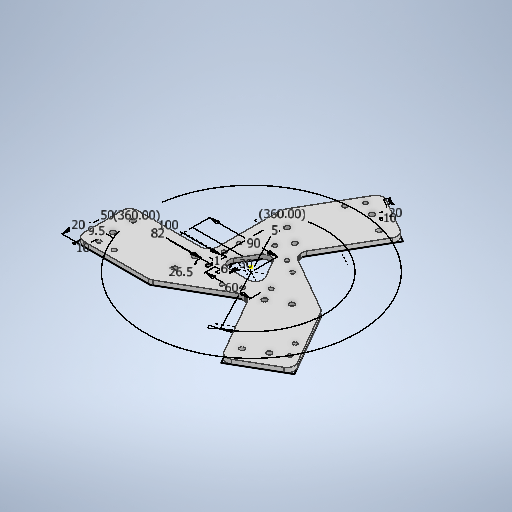
# Autodesk Inventor part: RT_FRM_MC_V3_MotorBase
Saved by Autodesk Inventor 2025.3 (Build 293356000, 356)
## iProperties
Created: 2026-09-20
Part Number: RT_FRM_MC_V3_MotorBase
Material: Generic
Document SubType Name: Modeling
Designer: louis
Density: 1 g/cm^3
Appearance: Default
Author: louis
Autodesk Inventor part; units mm, degrees
ref_plane "YZ Plane" through (0, 0, 0) normal (1, 0, 0) x (0, 1, 0)
ref_plane "XZ Plane" through (0, 0, 0) normal (0, 1, 0) x (-1, 0, 0)
ref_plane "XY Plane" through (0, 0, 0) normal (0, 0, 1) x (1, 0, 0)
sketch "Sketch1" plane through (0, 0, 0) normal (0, 0, 1) x (1, 0, 0)
  line L0 (-131, -26) -> (-49, -26) construction
  line L1 (-49, -26) -> (-49, -52.5) construction
  line L2 (-49, -52.5) -> (-131, -52.5) construction
  line L3 (-131, -52.5) -> (-131, -26) construction
  line L4 (-90, -26) -> (-90, 12) construction
  line L5 (-140, -12) -> (-40, -12) construction
  line L6 (-40, -12) -> (-40, -62) construction
  line L7 (-40, -62) -> (-140, -62) construction
  line L8 (-140, -62) -> (-140, -12) construction
  line L9 (-140, -18) -> (-40, -18) construction
  line L10 (-90, -12) -> (-90, 12) construction
  line L11 (0, 0) -> (-90, 0) construction
  line L12 (-30, -17.3205) -> (0, 34.641)
  line L13 (0, 34.641) -> (30, -17.3205)
  line L14 (30, -17.3205) -> (-30, -17.3205)
  line L15 (0, -17.3205) -> (0, 34.641) construction
  line L16 (-15, 8.6603) -> (30, -17.3205) construction
  line L17 (15, 8.6603) -> (-30, -17.3205) construction
  line L18 (80.3923, -115.2436) -> (30.3923, -28.641) construction
  line L19 (123.6936, -90.2436) -> (80.3923, -115.2436) construction
  line L20 (73.6936, -3.641) -> (123.6936, -90.2436) construction
  line L21 (30.3923, -28.641) -> (73.6936, -3.641) construction
  line L22 (67.5167, -64.9423) -> (34.6077, -83.9423) construction
  line L23 (59.6077, 127.2436) -> (9.6077, 40.641) construction
  line L24 (16.3064, 152.2436) -> (59.6077, 127.2436) construction
  line L25 (-33.6936, 65.641) -> (16.3064, 152.2436) construction
  line L26 (9.6077, 40.641) -> (-33.6936, 65.641) construction
  line L27 (22.4833, 90.9423) -> (55.3923, 71.9423) construction
  line L28 (3.9859, 170.9038) -> (-45, 86.0577)
  line L29 (-45, 86.0577) -> (-45, -11)
  line L30 (-45, -11) -> (-150, -11)
  line L31 (-150, -11) -> (-150, -82)
  line L32 (-52.0282, -82) -> (32.0263, -33.4711)
  line L33 (84.5263, -124.4038) -> (146.0141, -88.9038)
  line L34 (32.0263, -33.4711) -> (84.5263, -124.4038)
  line L35 (-150, -82) -> (-52.0282, -82)
  line L36 (97.0282, -4.0577) -> (12.9737, 44.4711)
  line L37 (65.4737, 135.4038) -> (3.9859, 170.9038)
  line L38 (12.9737, 44.4711) -> (65.4737, 135.4038)
  line L39 (146.0141, -88.9038) -> (97.0282, -4.0577)
  point P0 (-90, -18)
  point P1 (55.3923, -71.9423)
  point P2 (85.5885, -112.2436)
  point P3 (35.5885, -25.641)
  point P4 (110.9663, -87.1993)
  point P5 (69.9663, -16.1852)
  point P6 (47.0167, -29.4352)
  point P7 (88.0167, -100.4493)
  point P8 (34.6077, 83.9423)
  point P9 (54.4115, 130.2436)
  point P10 (4.4115, 43.641)
  point P11 (20.0337, 139.6993)
  point P12 (-20.9663, 68.6852)
  point P13 (1.9833, 55.4352)
  point P14 (42.9833, 126.4493)
  point P15 (3.9859, 170.9038)
  point P16 (-150, -82)
  point P17 (146.0141, -88.9038)
  dimension "d0" = 26.5
  dimension "d1" = 82
  dimension "d2" = 9.5
  dimension "d3" = 100
  dimension "d4" = 50
  dimension "d5" = 6
  dimension "d6" = 30
  dimension "d7" = 90
  dimension "d8" = 60
  dimension "d11" = 360
  dimension "d13" = 20
  dimension "d14" = 1
  dimension "d15" = 10
  dimension "d16" = 20
  dimension "d17" = 10
  dimension "d18" = 5
  dimension "d21" = 360
  constraints: 80 end point, 9 point on line, 7 midpoint, 7 perpendicular, 4 coincident, 4 parallel, 3 horizontal, 2 equal length, 2 vertical, 1 collinear, 84 other
  measures "d0" distance of L0.end L1.end
  measures "d1" distance of L0.start L0.end
  measures "d2" distance from line of L7 L2.end
  measures "d3" distance of L5.start L5.end
  measures "d4" distance of L7.end L5.start
  measures "d5" distance between parallel lines of L5 L9
  measures "d6" distance of L4.end point (-90, -18)
  measures "d7" distance from line of L11.start L4
  measures "d8" distance of L13.end L12.start
  measures "d13" distance between parallel lines of L25 L28
  measures "d14" distance between parallel lines of L5 L30
  measures "d15" distance between parallel lines of L8 L31
  measures "d16" distance from line of L31.end L7
  measures "d17" distance from line of L28.start L24
  measures "d18" distance between parallel lines of L29 L6
extrude "Extrusion1" add sketch "Sketch1" along normal blind 6
hole "Hole1" at (-131, -26, 0) at (-49, -26, 0) at (-49, -52.5, 0) at (-131, -52.5, 0) at (110.9663, -87.1993, 0) at (69.9663, -16.1852, 0) at (47.0167, -29.4352, 0) at (88.0167, -100.4493, 0) at (20.0337, 139.6993, 0) at (-20.9663, 68.6852, 0) at (1.9833, 55.4352, 0) at (42.9833, 126.4493, 0) direction (0, 0, 1) diameter 6.6 end through all clearance for "Socket Head Cap Screw" size "M6" standard "Ansi Metric M Profile"
chamfer "Chamfer1" distance 7.5 angle 45 3 edges at (32.0263, -33.4711, 3) (12.9737, 44.4711, 3) (-45, -11, 3)
fillet "Fillet1" radius 10 6 edges at (84.5263, -124.4038, 3) (146.0141, -88.9038, 3) (-52.0282, -82, 3) (35.7763, -39.9663, 3) (25.5311, -37.2211, 3) (30, -17.3205, 3)
pattern_circular "Circular Pattern1" count 3 over 360 about axis through (0, 0, -10) along (0, 0, 1) of "Fillet1"
sketch "Sketch2" plane through (0, 0, 6) normal (0, 0, 1) x (1, 0, 0)
  point P0 (0, 0)
sketch "Sketch3" plane through (0, 0, 0) normal (0, 0, -1) x (-1, 0, 0)
  line L0 (-94.7077, -2.718) -> (-23.0561, 38.6501) projected
  line L1 (-141.0141, -80.2436) -> (-98.3679, -6.3782) projected
  line L2 (-93.1865, -119.4038) -> (-137.3538, -93.9038) projected
  line L3 (-8.6603, 19.641) -> (-21.3397, -2.3205) projected
  line L4 (-37.8473, -43.5535) -> (-79.5263, -115.7436) projected
  line L5 (-18.7948, 54.5535) -> (-60.4737, 126.7436) projected
  line L6 (-123.6936, -90.2436) -> (-113.6936, -72.923)
  line L7 (-113.6936, -72.923) -> (-131.0141, -62.923)
  line L8 (-131.0141, -62.923) -> (-141.0141, -80.2436)
  line L9 (-141.0141, -80.2436) -> (-123.6936, -90.2436)
  line L10 (-123.6936, -90.2436) -> (-131.0141, -62.923) construction
  line L11 (-113.6936, -72.923) -> (-141.0141, -80.2436) construction
  point P0 (0, 0)
  point P1 (-117.3538, -59.2628)
  point P2 (-127.3538, -76.5833)
  point P3 (-33.9545, 20.8109)
  point P4 (-16.634, 30.8109)
  point P5 (-38.6603, -12.3205)
  dimension "d39" = 10
  dimension "d40" = 10
  dimension "d41" = 20
  dimension "d42" = 20
  dimension "d43" = 10
  dimension "d44" = 10
  dimension "d46" = 10
  dimension "d47" = 20
  dimension "d49" = 120
  dimension "d50" = 30
  dimension "d58" = 20
  dimension "d59" = 20
  constraints: 12 end point, 2 midpoint, 2 parallel, 1 collinear, 1 perpendicular
  measures "d39" distance from line of L0 point (-33.954, 20.811)
  measures "d40" distance from line of L0 point (-16.634, 30.811)
  measures "d41" distance of point (-16.634, 30.811) point (-33.954, 20.811)
  measures "d42" distance of point (-127.354, -76.583) point (-117.354, -59.263)
  measures "d43" distance from line of L1 point (-117.354, -59.263)
  measures "d44" distance from line of L1 point (-127.354, -76.583)
  measures "d46" distance from line of L3 point (-38.66, -12.321)
  measures "d47" distance from line of L2 point (-127.354, -76.583)
  measures "d49" distance from line of L2 point (-38.66, -12.321)
  measures "d50" distance from line of L5 point (-33.954, 20.811)
  measures "d58" distance of L6.end L7.end
  measures "d59" distance of L6.start L6.end
hole "Hole2" at (38.6603, -12.3205, 0) at (33.9545, 20.8109, 0) at (16.634, 30.8109, 0) at (127.3538, -76.5833, 0) at (117.3538, -59.2628, 0) direction (0, 0, 1) diameter 5.5 end through all clearance for "Socket Head Cap Screw" size "M5" standard "Ansi Metric M Profile"
pattern_circular "Circular Pattern2" count 3 over 360 about axis through (0, 0, -10) along (0, 0, 1) of "Hole2"
equation "\"d44\" = d43"
body "Solid1"
